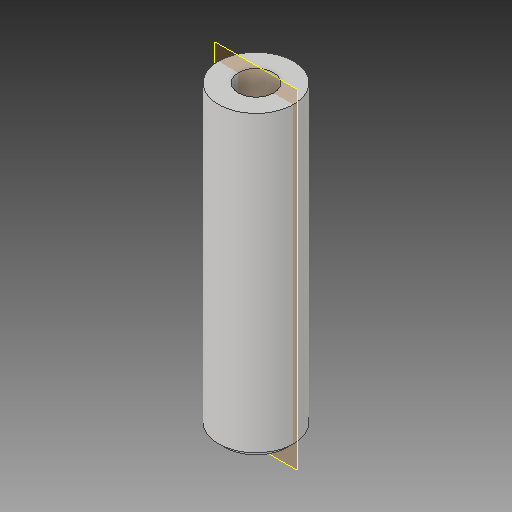
# Autodesk Inventor part: barrel
Saved by Autodesk Inventor 2018 (Build 220112000, 112)
## iProperties
Created: 2017-05-30
Part Number: barrel
Material: Generic
Document SubType Name: Modeling
Designer: m207653
Density: 1 g/cm^3
Appearance: Default
Author: m207653
Autodesk Inventor part; units mm, degrees
ref_plane "YZ Plane" through (0, 0, 0) normal (1, 0, 0) x (0, 1, 0)
ref_plane "XZ Plane" through (0, 0, 0) normal (0, 1, 0) x (-1, 0, 0)
sketch "Sketch1" plane through (0, 0, 0) normal (0, 1, 0) x (-1, 0, 0)
  circle A0 centre (0, 0) radius 25
  circle A1 centre (0, 0) radius 11.75
  dimension "d0" = 50
  dimension "d1" = 23.5
  constraints: 2 centre point, 2 coincident
  measures "d0" diameter of A0
  measures "d1" diameter of A1
extrude "Extrusion1" add sketch "Sketch1" along normal blind 200
chamfer "Chamfer1" distance 4 angle 45 1 edges at (25, 0, 0)
body "Solid1"
